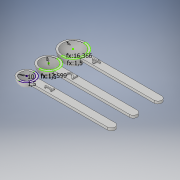
# Autodesk Inventor part: Pigmentlöffel
Saved by Autodesk Inventor 2018.2 (Build 222227000, 227)
## iProperties
Created: 2018-01-23
Part Number: Pigmentlöffel
Material: Generisch
Document SubType Name: Modeling
Designer: JochenAlt
Density: 1 g/cm^3
Appearance: Vorgabe
Author: JochenAlt
Autodesk Inventor part; units mm, degrees
ref_plane "XZ Plane" through (0, 0, 0) normal (0, 1, 0) x (-1, 0, 0)
ref_plane "XY Plane" through (0, 0, 0) normal (0, 0, 1) x (1, 0, 0)
sketch "Skizze1" plane through (0, 0, 0) normal (0, 0, 1) x (1, 0, 0)
  arc A0 (0, -5) -> (0, 5) centre (0, 0) ccw
  arc A1 (0, -6.5) -> (0, 6.5) centre (0, 0) ccw
  line L0 (0, -6.5) -> (0, -5)
  line L1 (0, 5) -> (0, 6.5)
  arc A2 (0, 11.07) -> (0, 23.669) centre (0, 17.3695) ccw
  arc A3 (0, 9.57) -> (0, 25.169) centre (0, 17.3695) ccw
  arc A4 (0, 28.5978) -> (0, 44.9639) centre (0, 36.7809) ccw
  arc A5 (0, 27.0978) -> (0, 46.4639) centre (0, 36.7809) ccw
  line L2 (0, 44.9639) -> (0, 46.4639)
  line L3 (0, 27.0978) -> (0, 28.5978)
  line L4 (0, 9.57) -> (0, 11.07)
  line L5 (0, 23.669) -> (0, 25.169)
  dimension "d0" = 10
  dimension "d8" = 1.5
  dimension "d9" = 12.599
  dimension "d10" = 1.5
  dimension "d11" = 16.3661
  dimension "d12" = 1.5
  constraints: 12 end point, 12 point on circle, 6 centre point, 6 vertical, 4 coincident
  measures "d0" diameter of A0
  measures "d8" radial gap between concentric circles of A1 A0
  measures "d9" diameter of A2
  measures "d10" radial gap between concentric circles of A3 A2
  measures "d11" diameter of A4
  measures "d12" radial gap between concentric circles of A5 A4
revolve "Umdrehung1" add sketch "Skizze1" angle 180 about axis through (0, -6.5, 0) along (0, 1, 0) contours A0 L1 A1 L0
revolve "Umdrehung2" add sketch "Skizze1" angle 180 about axis through (0, 9.57, 0) along (0, 1, 0) contours A2 L5 A3 L4
revolve "Umdrehung3" add sketch "Skizze1" angle 180 about axis through (0, 27.0978, 0) along (0, 1, 0) contours A4 L2 A5 L3
ref_plane "Arbeitsebene1" through (70, 0, 0) normal (1, 0, 0) x (0, 1, 0)
sketch "Skizze3" plane through (70, 0, 0) normal (1, 0, 0) x (0, 1, 0)
  line L0 (-5, 0) -> (5, 0) projected
  line L1 (-3, 0) -> (3, 0)
  line L2 (3, 0) -> (3, -2)
  line L3 (3, -2) -> (-3, -2)
  line L4 (-3, -2) -> (-3, 0)
  line L5 (14.3695, 0) -> (20.3695, 0)
  line L6 (20.3695, 0) -> (20.3695, -2)
  line L7 (20.3695, -2) -> (14.3695, -2)
  line L8 (14.3695, -2) -> (14.3695, 0)
  line L9 (33.7809, 0) -> (39.7809, 0)
  line L10 (39.7809, 0) -> (39.7809, -2)
  line L11 (39.7809, -2) -> (33.7809, -2)
  line L12 (33.7809, -2) -> (33.7809, 0)
  line L13 (25.169, 0) -> (9.57, 0) construction
  line L14 (46.4639, 0) -> (27.0978, 0) construction
  arc A0 (-5, 0) -> (5, 0) centre (0, 0) ccw construction
  line L15 (6.5, 0) -> (-6.5, 0) construction
  line L16 (0, 1.9354) -> (0, -11.6125) construction
  line L17 (-17.0928, 0) -> (57.0567, 0) construction
  line L18 (36.7809, 0) -> (36.7809, -9.6771) construction
  line L19 (17.3695, 0) -> (17.3695, -7.848) construction
  dimension "d16" = 2
  dimension "d17" = 6
  dimension "d21" = 6
  dimension "d22" = 6
  constraints: 28 end point, 6 parallel, 3 coincident, 3 horizontal, 3 perpendicular, 3 point on line, 2 collinear, 2 vertical, 4 other
  measures "d16" distance of the line from the sketch origin of L3
  measures "d17" distance between parallel lines of L2 L4
  measures "d21" distance between parallel lines of L6 L8
  measures "d22" distance between parallel lines of L10 L12
extrude "Extrusion2" add sketch "Skizze3" against normal up to next
fillet "Rundung1" radius 3 6 edges at (70, 3, -1) (70, -3, -1) (70, 14.3695, -1) (70, 20.3695, -1) (70, 33.7809, -1) (70, 39.7809, -1)
sketch "Skizze5" plane through (0, 0, 0) normal (0, 0, 1) x (1, 0, 0)
  line L0 (20.5874, 1.818) -> (20.5874, -1.1578)
  line L1 (20.5874, -1.1578) -> (19.9646, -1.1578)
  line L2 (19.9646, -1.1578) -> (19.9646, -0.0505)
  line L3 (19.9646, -0.0505) -> (15.8765, -0.0505)
  line L4 (15.8765, -0.0505) -> (15.8765, -1.1578)
  line L5 (15.8765, -1.1578) -> (15.3179, -1.1578)
  spline S0 degree 2 poles (15.3179, -1.1578) (15.3179, -0.53) (14.962, 0.0632) (14.4677, 0.1027) knots 0 0 0 1 2 2 2
  line L6 (14.4677, 0.1027) -> (14.4677, 0.7354)
  line L7 (14.4677, 0.7354) -> (19.9646, 0.7354)
  line L8 (19.9646, 0.7354) -> (19.9646, 1.818)
  line L9 (19.9646, 1.818) -> (20.5874, 1.818)
  line L10 (20.8624, 19.5576) -> (20.8624, 15.7958)
  line L11 (20.8624, 15.7958) -> (19.9973, 15.7958)
  spline S1 degree 2 poles (19.9973, 15.7958) (19.6167, 16.2012) (18.9098, 16.9229) (18.5292, 17.2689) knots 0 0 0 1 2 2 2
  spline S2 degree 2 poles (18.5292, 17.2689) (17.763, 17.9659) (16.8435, 18.4751) (16.3541, 18.4751) knots 0 0 0 1 2 2 2
  spline S3 degree 2 poles (16.3541, 18.4751) (16.0971, 18.4751) (15.7115, 18.3169) (15.5879, 18.1735) knots 0 0 0 1 2 2 2
  spline S4 degree 2 poles (15.5879, 18.1735) (15.4643, 18.0302) (15.3408, 17.6545) (15.3408, 17.4271) knots 0 0 0 1 2 2 2
  spline S5 degree 2 poles (15.3408, 17.4271) (15.3408, 17.2096) (15.4495, 16.7647) (15.5335, 16.562) knots 0 0 0 1 2 2 2
  spline S6 degree 2 poles (15.5335, 16.562) (15.6027, 16.389) (15.8005, 16.0677) (15.8697, 15.9688) knots 0 0 0 1 2 2 2
  line L12 (15.8697, 15.9688) -> (15.8697, 15.9243)
  line L13 (15.8697, 15.9243) -> (14.9997, 15.9243)
  spline S7 degree 2 poles (14.9997, 15.9243) (14.8761, 16.1764) (14.6339, 17.0811) (14.6339, 17.4864) knots 0 0 0 1 2 2 2
  spline S8 degree 2 poles (14.6339, 17.4864) (14.6339, 18.3416) (15.5385, 19.3055) (16.3096, 19.3055) knots 0 0 0 1 2 2 2
  spline S9 degree 2 poles (16.3096, 19.3055) (16.6705, 19.3055) (17.2736, 19.1375) (17.5306, 18.9892) knots 0 0 0 1 2 2 2
  spline S10 degree 2 poles (17.5306, 18.9892) (17.7976, 18.8409) (18.3215, 18.4108) (18.5737, 18.1735) knots 0 0 0 1 2 2 2
  spline S11 degree 2 poles (18.5737, 18.1735) (18.9938, 17.7879) (19.8935, 16.8438) (20.1555, 16.562) knots 0 0 0 1 2 2 2
  line L14 (20.1555, 16.562) -> (20.1555, 19.5576)
  line L15 (20.1555, 19.5576) -> (20.8624, 19.5576)
  line L16 (18.4703, 38.8851) -> (18.4703, 38.1585)
  line L17 (18.4703, 38.1585) -> (20.5663, 38.1585)
  line L18 (20.5663, 38.1585) -> (20.5663, 37.3725)
  line L19 (20.5663, 37.3725) -> (18.4703, 37.3725)
  line L20 (18.4703, 37.3725) -> (18.4703, 34.6784)
  line L21 (18.4703, 34.6784) -> (17.6102, 34.6784)
  line L22 (17.6102, 34.6784) -> (14.4663, 37.4071)
  line L23 (14.4663, 37.4071) -> (14.4663, 38.1585)
  line L24 (14.4663, 38.1585) -> (17.8129, 38.1585)
  line L25 (17.8129, 38.1585) -> (17.8129, 38.8851)
  line L26 (17.8129, 38.8851) -> (18.4703, 38.8851)
  line L27 (17.8129, 37.3725) -> (15.4302, 37.3725)
  line L28 (15.4302, 37.3725) -> (17.8129, 35.321)
  line L29 (17.8129, 35.321) -> (17.8129, 37.3725)
  point P0 (0, 0)
  point P1 (14.4677, -2.0822)
  point P2 (17.5163, 34.5153)
  point P3 (17.7481, 15.3509)
  constraints: 3 other
extrude "Extrusion4" add sketch "Skizze5" along normal blind 0.6
equation "\"d9\" = 1.2599 * d0"
equation "\"d10\" = d8"
equation "\"d11\" = 1.299 * d9"
equation "\"d12\" = d10"
equation "\"d21\" = d17"
equation "\"d22\" = d17"
